Autodesk Fusion 360 part; units mm, degrees
(part 3 of 3)
  arc A275 (-147.4938, 83.5375) -> (-146.4938, 82.5375) centre (-146.4938, 83.5375) ccw
  line L265 (-147.4938, 83.5375) -> (-147.4938, 95.5375)
  arc A276 (-146.4938, 96.5375) -> (-147.4938, 95.5375) centre (-146.4938, 95.5375) ccw
  line L266 (-146.4938, 96.5375) -> (-134.4938, 96.5375)
  arc A277 (-133.4938, 95.5375) -> (-134.4938, 96.5375) centre (-134.4938, 95.5375) ccw
  line L267 (-133.4938, 95.5375) -> (-133.4938, 83.5375)
  arc A278 (-351.1875, 63.4875) -> (-350.1875, 64.4875) centre (-351.1875, 64.4875) ccw
  line L268 (-351.1875, 63.4875) -> (-363.1875, 63.4875)
  arc A279 (-364.1875, 64.4875) -> (-363.1875, 63.4875) centre (-363.1875, 64.4875) ccw
  line L269 (-364.1875, 64.4875) -> (-364.1875, 76.4875)
  arc A280 (-363.1875, 77.4875) -> (-364.1875, 76.4875) centre (-363.1875, 76.4875) ccw
  line L270 (-363.1875, 77.4875) -> (-351.1875, 77.4875)
  arc A281 (-350.1875, 76.4875) -> (-351.1875, 77.4875) centre (-351.1875, 76.4875) ccw
  line L271 (-350.1875, 76.4875) -> (-350.1875, 64.4875)
  arc A282 (-3.525, 82.5375) -> (-2.525, 83.5375) centre (-3.525, 83.5375) ccw
  line L272 (-3.525, 82.5375) -> (-15.525, 82.5375)
  arc A283 (-16.525, 83.5375) -> (-15.525, 82.5375) centre (-15.525, 83.5375) ccw
  line L273 (-16.525, 83.5375) -> (-16.525, 95.5375)
  arc A284 (-15.525, 96.5375) -> (-16.525, 95.5375) centre (-15.525, 95.5375) ccw
  line L274 (-15.525, 96.5375) -> (-3.525, 96.5375)
  arc A285 (-2.525, 95.5375) -> (-3.525, 96.5375) centre (-3.525, 95.5375) ccw
  line L275 (-2.525, 95.5375) -> (-2.525, 83.5375)
  arc A286 (-246.4125, 63.4875) -> (-245.4125, 64.4875) centre (-246.4125, 64.4875) ccw
  line L276 (-246.4125, 63.4875) -> (-258.4125, 63.4875)
  arc A287 (-259.4125, 64.4875) -> (-258.4125, 63.4875) centre (-258.4125, 64.4875) ccw
  line L277 (-259.4125, 64.4875) -> (-259.4125, 76.4875)
  arc A288 (-258.4125, 77.4875) -> (-259.4125, 76.4875) centre (-258.4125, 76.4875) ccw
  line L278 (-258.4125, 77.4875) -> (-246.4125, 77.4875)
  arc A289 (-245.4125, 76.4875) -> (-246.4125, 77.4875) centre (-246.4125, 76.4875) ccw
  line L279 (-245.4125, 76.4875) -> (-245.4125, 64.4875)
  arc A290 (-132.1125, 63.4875) -> (-131.1125, 64.4875) centre (-132.1125, 64.4875) ccw
  line L280 (-132.1125, 63.4875) -> (-144.1125, 63.4875)
  arc A291 (-145.1125, 64.4875) -> (-144.1125, 63.4875) centre (-144.1125, 64.4875) ccw
  line L281 (-145.1125, 64.4875) -> (-145.1125, 76.4875)
  arc A292 (-144.1125, 77.4875) -> (-145.1125, 76.4875) centre (-144.1125, 76.4875) ccw
  line L282 (-144.1125, 77.4875) -> (-132.1125, 77.4875)
  arc A293 (-131.1125, 76.4875) -> (-132.1125, 77.4875) centre (-132.1125, 76.4875) ccw
  line L283 (-131.1125, 76.4875) -> (-131.1125, 64.4875)
  arc A294 (-208.3125, 63.4875) -> (-207.3125, 64.4875) centre (-208.3125, 64.4875) ccw
  line L284 (-208.3125, 63.4875) -> (-220.3125, 63.4875)
  arc A295 (-221.3125, 64.4875) -> (-220.3125, 63.4875) centre (-220.3125, 64.4875) ccw
  line L285 (-221.3125, 64.4875) -> (-221.3125, 76.4875)
  arc A296 (-220.3125, 77.4875) -> (-221.3125, 76.4875) centre (-220.3125, 76.4875) ccw
  line L286 (-220.3125, 77.4875) -> (-208.3125, 77.4875)
  arc A297 (-207.3125, 76.4875) -> (-208.3125, 77.4875) centre (-208.3125, 76.4875) ccw
  line L287 (-207.3125, 76.4875) -> (-207.3125, 64.4875)
  arc A298 (-265.4625, 63.4875) -> (-264.4625, 64.4875) centre (-265.4625, 64.4875) ccw
  line L288 (-265.4625, 63.4875) -> (-277.4625, 63.4875)
  arc A299 (-278.4625, 64.4875) -> (-277.4625, 63.4875) centre (-277.4625, 64.4875) ccw
  line L289 (-278.4625, 64.4875) -> (-278.4625, 76.4875)
  arc A300 (-277.4625, 77.4875) -> (-278.4625, 76.4875) centre (-277.4625, 76.4875) ccw
  line L290 (-277.4625, 77.4875) -> (-265.4625, 77.4875)
  arc A301 (-264.4625, 76.4875) -> (-265.4625, 77.4875) centre (-265.4625, 76.4875) ccw
  line L291 (-264.4625, 76.4875) -> (-264.4625, 64.4875)
  line L292 (-188.2625, 76.4875) -> (-188.2625, 64.4875)
  arc A302 (-189.2625, 63.4875) -> (-188.2625, 64.4875) centre (-189.2625, 64.4875) ccw
  line L293 (-189.2625, 63.4875) -> (-201.2625, 63.4875)
  arc A303 (-202.2625, 64.4875) -> (-201.2625, 63.4875) centre (-201.2625, 64.4875) ccw
  line L294 (-202.2625, 64.4875) -> (-202.2625, 76.4875)
  arc A304 (-201.2625, 77.4875) -> (-202.2625, 76.4875) centre (-201.2625, 76.4875) ccw
  line L295 (-201.2625, 77.4875) -> (-189.2625, 77.4875)
  arc A305 (-188.2625, 76.4875) -> (-189.2625, 77.4875) centre (-189.2625, 76.4875) ccw
  arc A306 (-227.3625, 63.4875) -> (-226.3625, 64.4875) centre (-227.3625, 64.4875) ccw
  line L296 (-227.3625, 63.4875) -> (-239.3625, 63.4875)
  arc A307 (-240.3625, 64.4875) -> (-239.3625, 63.4875) centre (-239.3625, 64.4875) ccw
  line L297 (-240.3625, 64.4875) -> (-240.3625, 76.4875)
  arc A308 (-239.3625, 77.4875) -> (-240.3625, 76.4875) centre (-239.3625, 76.4875) ccw
  line L298 (-239.3625, 77.4875) -> (-227.3625, 77.4875)
  arc A309 (-226.3625, 76.4875) -> (-227.3625, 77.4875) centre (-227.3625, 76.4875) ccw
  line L299 (-226.3625, 76.4875) -> (-226.3625, 64.4875)
  arc A310 (-170.2125, 63.4875) -> (-169.2125, 64.4875) centre (-170.2125, 64.4875) ccw
  line L300 (-170.2125, 63.4875) -> (-182.2125, 63.4875)
  arc A311 (-183.2125, 64.4875) -> (-182.2125, 63.4875) centre (-182.2125, 64.4875) ccw
  line L301 (-183.2125, 64.4875) -> (-183.2125, 76.4875)
  arc A312 (-182.2125, 77.4875) -> (-183.2125, 76.4875) centre (-182.2125, 76.4875) ccw
  line L302 (-182.2125, 77.4875) -> (-170.2125, 77.4875)
  arc A313 (-169.2125, 76.4875) -> (-170.2125, 77.4875) centre (-170.2125, 76.4875) ccw
  line L303 (-169.2125, 76.4875) -> (-169.2125, 64.4875)
  arc A314 (-76.0563, 64.4875) -> (-75.0563, 63.4875) centre (-75.0563, 64.4875) ccw
  line L304 (-76.0563, 64.4875) -> (-76.0563, 76.4875)
  arc A315 (-75.0563, 77.4875) -> (-76.0563, 76.4875) centre (-75.0563, 76.4875) ccw
  line L305 (-75.0563, 77.4875) -> (-63.0562, 77.4875)
  arc A316 (-62.0563, 76.4875) -> (-63.0562, 77.4875) centre (-63.0562, 76.4875) ccw
  line L306 (-62.0563, 76.4875) -> (-62.0563, 64.4875)
  arc A317 (-63.0562, 63.4875) -> (-62.0563, 64.4875) centre (-63.0562, 64.4875) ccw
  line L307 (-63.0562, 63.4875) -> (-75.0563, 63.4875)
  line L308 (-112.0625, 76.4875) -> (-112.0625, 64.4875)
  arc A318 (-113.0625, 63.4875) -> (-112.0625, 64.4875) centre (-113.0625, 64.4875) ccw
  line L309 (-113.0625, 63.4875) -> (-125.0625, 63.4875)
  arc A319 (-126.0625, 64.4875) -> (-125.0625, 63.4875) centre (-125.0625, 64.4875) ccw
  line L310 (-126.0625, 64.4875) -> (-126.0625, 76.4875)
  arc A320 (-125.0625, 77.4875) -> (-126.0625, 76.4875) centre (-125.0625, 76.4875) ccw
  line L311 (-125.0625, 77.4875) -> (-113.0625, 77.4875)
  arc A321 (-112.0625, 76.4875) -> (-113.0625, 77.4875) centre (-113.0625, 76.4875) ccw
  arc A322 (-164.1625, 64.4875) -> (-163.1625, 63.4875) centre (-163.1625, 64.4875) ccw
  line L312 (-164.1625, 64.4875) -> (-164.1625, 76.4875)
  arc A323 (-163.1625, 77.4875) -> (-164.1625, 76.4875) centre (-163.1625, 76.4875) ccw
  line L313 (-163.1625, 77.4875) -> (-151.1625, 77.4875)
  arc A324 (-150.1625, 76.4875) -> (-151.1625, 77.4875) centre (-151.1625, 76.4875) ccw
  line L314 (-150.1625, 76.4875) -> (-150.1625, 64.4875)
  arc A325 (-151.1625, 63.4875) -> (-150.1625, 64.4875) centre (-151.1625, 64.4875) ccw
  line L315 (-151.1625, 63.4875) -> (-163.1625, 63.4875)
  arc A326 (-3.525, 63.4875) -> (-2.525, 64.4875) centre (-3.525, 64.4875) ccw
  line L316 (-3.525, 63.4875) -> (-15.525, 63.4875)
  arc A327 (-16.525, 64.4875) -> (-15.525, 63.4875) centre (-15.525, 64.4875) ccw
  line L317 (-16.525, 64.4875) -> (-16.525, 76.4875)
  arc A328 (-15.525, 77.4875) -> (-16.525, 76.4875) centre (-15.525, 76.4875) ccw
  line L318 (-15.525, 77.4875) -> (-3.525, 77.4875)
  arc A329 (-2.525, 76.4875) -> (-3.525, 77.4875) centre (-3.525, 76.4875) ccw
  line L319 (-2.525, 76.4875) -> (-2.525, 64.4875)
  arc A330 (-94.0125, 63.4875) -> (-93.0125, 64.4875) centre (-94.0125, 64.4875) ccw
  line L320 (-94.0125, 63.4875) -> (-106.0125, 63.4875)
  arc A331 (-107.0125, 64.4875) -> (-106.0125, 63.4875) centre (-106.0125, 64.4875) ccw
  line L321 (-107.0125, 64.4875) -> (-107.0125, 76.4875)
  arc A332 (-106.0125, 77.4875) -> (-107.0125, 76.4875) centre (-106.0125, 76.4875) ccw
  line L322 (-106.0125, 77.4875) -> (-94.0125, 77.4875)
  arc A333 (-93.0125, 76.4875) -> (-94.0125, 77.4875) centre (-94.0125, 76.4875) ccw
  line L323 (-93.0125, 76.4875) -> (-93.0125, 64.4875)
  arc A334 (-54.6183, 64.4875) -> (-53.6183, 65.4875) centre (-54.6183, 65.4875) ccw
  line L324 (-54.6183, 64.4875) -> (-59.6183, 64.4875)
  arc A335 (-60.6183, 65.4875) -> (-59.6183, 64.4875) centre (-59.6183, 65.4875) ccw
  line L325 (-60.6183, 65.4875) -> (-60.6183, 78.4875)
  arc A336 (-59.6183, 79.4875) -> (-60.6183, 78.4875) centre (-59.6183, 78.4875) ccw
  line L326 (-59.6183, 79.4875) -> (-54.6183, 79.4875)
  arc A337 (-53.6183, 78.4875) -> (-54.6183, 79.4875) centre (-54.6183, 78.4875) ccw
  line L327 (-53.6183, 78.4875) -> (-53.6183, 65.4875)
  arc A338 (-78.4942, 64.4875) -> (-77.4942, 65.4875) centre (-78.4942, 65.4875) ccw
  line L328 (-78.4942, 64.4875) -> (-83.4942, 64.4875)
  arc A339 (-84.4942, 65.4875) -> (-83.4942, 64.4875) centre (-83.4942, 65.4875) ccw
  line L329 (-84.4942, 65.4875) -> (-84.4942, 78.4875)
  arc A340 (-83.4942, 79.4875) -> (-84.4942, 78.4875) centre (-83.4942, 78.4875) ccw
  line L330 (-83.4942, 79.4875) -> (-78.4942, 79.4875)
  arc A341 (-77.4942, 78.4875) -> (-78.4942, 79.4875) centre (-78.4942, 78.4875) ccw
  line L331 (-77.4943, 78.4875) -> (-77.4943, 65.4875)
  arc A342 (-351.1875, 44.4375) -> (-350.1875, 45.4375) centre (-351.1875, 45.4375) ccw
  line L332 (-351.1875, 44.4375) -> (-363.1875, 44.4375)
  arc A343 (-364.1875, 45.4375) -> (-363.1875, 44.4375) centre (-363.1875, 45.4375) ccw
  line L333 (-364.1875, 45.4375) -> (-364.1875, 57.4375)
  arc A344 (-363.1875, 58.4375) -> (-364.1875, 57.4375) centre (-363.1875, 57.4375) ccw
  line L334 (-363.1875, 58.4375) -> (-351.1875, 58.4375)
  arc A345 (-350.1875, 57.4375) -> (-351.1875, 58.4375) centre (-351.1875, 57.4375) ccw
  line L335 (-350.1875, 57.4375) -> (-350.1875, 45.4375)
  arc A346 (-22.575, 63.4875) -> (-21.575, 64.4875) centre (-22.575, 64.4875) ccw
  line L336 (-22.575, 63.4875) -> (-34.575, 63.4875)
  arc A347 (-35.575, 64.4875) -> (-34.575, 63.4875) centre (-34.575, 64.4875) ccw
  line L337 (-35.575, 64.4875) -> (-35.575, 76.4875)
  arc A348 (-34.575, 77.4875) -> (-35.575, 76.4875) centre (-34.575, 76.4875) ccw
  line L338 (-34.575, 77.4875) -> (-22.575, 77.4875)
  arc A349 (-21.575, 76.4875) -> (-22.575, 77.4875) centre (-22.575, 76.4875) ccw
  line L339 (-21.575, 76.4875) -> (-21.575, 64.4875)
  arc A350 (-198.7875, 44.4375) -> (-197.7875, 45.4375) centre (-198.7875, 45.4375) ccw
  line L340 (-198.7875, 44.4375) -> (-210.7875, 44.4375)
  arc A351 (-211.7875, 45.4375) -> (-210.7875, 44.4375) centre (-210.7875, 45.4375) ccw
  line L341 (-211.7875, 45.4375) -> (-211.7875, 57.4375)
  arc A352 (-210.7875, 58.4375) -> (-211.7875, 57.4375) centre (-210.7875, 57.4375) ccw
  line L342 (-210.7875, 58.4375) -> (-198.7875, 58.4375)
  arc A353 (-197.7875, 57.4375) -> (-198.7875, 58.4375) centre (-198.7875, 57.4375) ccw
  line L343 (-197.7875, 57.4375) -> (-197.7875, 45.4375)
  arc A354 (-321.3818, 45.4375) -> (-320.3818, 46.4375) centre (-321.3818, 46.4375) ccw
  line L344 (-321.3818, 45.4375) -> (-326.3818, 45.4375)
  arc A355 (-327.3818, 46.4375) -> (-326.3818, 45.4375) centre (-326.3818, 46.4375) ccw
  line L345 (-327.3818, 46.4375) -> (-327.3818, 59.4375)
  arc A356 (-326.3818, 60.4375) -> (-327.3818, 59.4375) centre (-326.3818, 59.4375) ccw
  line L346 (-326.3818, 60.4375) -> (-321.3818, 60.4375)
  arc A357 (-320.3818, 59.4375) -> (-321.3818, 60.4375) centre (-321.3818, 59.4375) ccw
  line L347 (-320.3818, 59.4375) -> (-320.3818, 46.4375)
  arc A358 (4.705, -8.8925) -> (12.705, -0.8925) centre (4.705, -0.8925) ccw
  line L348 (12.705, -0.8925) -> (12.705, 108.53)
  arc A359 (12.705, 108.53) -> (4.705, 116.53) centre (4.705, 108.53) ccw
  line L349 (4.705, 116.53) -> (-371.4175, 116.53)
  arc A360 (-371.4175, 116.53) -> (-379.4175, 108.53) centre (-371.4175, 108.53) ccw
  line L350 (-379.4175, 108.53) -> (-379.4175, -0.8925)
  arc A361 (-379.4175, -0.8925) -> (-371.4175, -8.8925) centre (-371.4175, -0.8925) ccw
  line L351 (-371.4175, -8.8925) -> (4.705, -8.8925)
  line L352 (1.644, 103.1073) -> (1.644, 5.1073)
  line L353 (-2.356, 1.1073) -> (-154.3938, 1.1073)
  line L354 (-364.356, 107.1073) -> (-2.356, 107.1073)
  arc A362 (1.644, 103.1073) -> (-2.356, 107.1073) centre (-2.356, 103.1073) ccw
  arc A363 (-2.356, 1.1073) -> (1.644, 5.1073) centre (-2.356, 5.1073) ccw
  line L355 (-169.3938, 1.1073) -> (-364.356, 1.1073)
  arc A364 (-368.356, 5.1073) -> (-364.356, 1.1073) centre (-364.356, 5.1073) ccw
  line L356 (-368.356, 5.1073) -> (-368.356, 103.1073)
  arc A365 (-364.356, 107.1073) -> (-368.356, 103.1073) centre (-364.356, 103.1073) ccw
  line L357 (-379.4175, -0.8925) -> (-379.4175, 108.53)
  arc A366 (-371.4175, 116.53) -> (-379.4175, 108.53) centre (-371.4175, 108.53) ccw
  line L358 (-371.4175, 116.53) -> (4.705, 116.53)
  arc A367 (12.705, 108.53) -> (4.705, 116.53) centre (4.705, 108.53) ccw
  line L359 (12.705, 108.53) -> (12.705, -0.8925)
  arc A368 (4.705, -8.8925) -> (12.705, -0.8925) centre (4.705, -0.8925) ccw
  line L360 (4.705, -8.8925) -> (-371.4175, -8.8925)
  arc A369 (-379.4175, -0.8925) -> (-371.4175, -8.8925) centre (-371.4175, -0.8925) ccw
  line L361 (-154.3938, 1.1073) -> (-169.3938, 1.1073)
  constraint coincident L353.end L361.start
  constraint coincident L355.start L361.end
extrude "Extrude11" add sketch "Sketch5" along normal blind 3 separate body contours A358 L348 A359 L349 A360 L350 A361 L351 L357 A366 L358 A367 L359 A368 L360 A369 makes body 4
equation "d113 = ( 4.6 / 2 ) * 1 mm"
